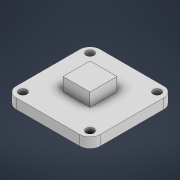
# Autodesk Inventor part: camera
Saved by Autodesk Inventor 2021 (Build 250183000, 183)
## iProperties
Created: 2020-12-29
Part Number: camera
Material: Generic
Document SubType Name: Modeling
Designer: Tomasz
Density: 1 g/cm^3
Appearance: Default
Author: Tomasz
Autodesk Inventor part; units mm, degrees
ref_plane "YZ Plane" through (0, 0, 0) normal (1, 0, 0) x (0, 1, 0)
ref_plane "XZ Plane" through (0, 0, 0) normal (0, 1, 0) x (-1, 0, 0)
ref_plane "XY Plane" through (0, 0, 0) normal (0, 0, 1) x (1, 0, 0)
sketch "Sketch1" plane through (0, 0, 0) normal (0, 1, 0) x (-1, 0, 0)
  line L0 (-9.5, 12.5) -> (9.5, 12.5)
  line L1 (12.5, 9.5) -> (12.5, -9.5)
  line L2 (9.5, -12.5) -> (-9.5, -12.5)
  line L3 (-12.5, -9.5) -> (-12.5, 9.5)
  line L4 (-12.5, 12.5) -> (12.5, -12.5) construction
  line L5 (12.5, 12.5) -> (-12.5, -12.5) construction
  line L6 (-10, -10) -> (10, -10) construction
  line L7 (10, -10) -> (10, 10) construction
  line L8 (10, 10) -> (-10, 10) construction
  line L9 (-10, 10) -> (-10, -10) construction
  line L10 (-10, -10) -> (10, 10) construction
  line L11 (10, -10) -> (-10, 10) construction
  circle A0 centre (10, 10) radius 1.2
  circle A1 centre (10, -10) radius 1.2
  circle A2 centre (-10, 10) radius 1.2
  circle A3 centre (-10, -10) radius 1.2
  arc A4 (12.5, 9.5) -> (9.5, 12.5) centre (9.5, 9.5) ccw
  arc A5 (9.5, -12.5) -> (12.5, -9.5) centre (9.5, -9.5) ccw
  arc A6 (-9.5, 12.5) -> (-12.5, 9.5) centre (-9.5, 9.5) ccw
  arc A7 (-12.5, -9.5) -> (-9.5, -12.5) centre (-9.5, -9.5) ccw
  point P0 (0, 0)
  dimension "d0" = 25
  dimension "d1" = 25
  dimension "d2" = 20
  dimension "d3" = 20
  dimension "d4" = 2.4
  dimension "d7" = 20
  dimension "d10" = 20
  dimension "d13" = 3
  constraints: 24 end point, 8 centre point, 8 point on circle, 8 point on line, 8 tangent, 4 midpoint, 4 parallel, 3 equal radius, 3 horizontal, 2 perpendicular, 1 coincident, 1 vertical, 6 other
  measures "d0" distance of L4.end L5.end
  measures "d1" distance of L5.start L4.end
  measures "d2" distance of L8.end L7.end
  measures "d3" distance of L7.end L6.end
  measures "d4" diameter of A0
  measures "d7" distance of A0.centre A1.centre
  measures "d10" distance of A0.centre A2.centre
  measures "d13" radius of A4
extrude "Extrusion1" add sketch "Sketch1" along normal blind 3
sketch "Sketch2" plane through (0, 3, 0) normal (0, 1, 0) x (1, 0, 0)
  line L0 (4, -4) -> (-4, -4)
  line L1 (-4, -4) -> (-4, 4)
  line L2 (-4, 4) -> (4, 4)
  line L3 (4, 4) -> (4, -4)
  line L4 (4, -4) -> (-4, 4) construction
  line L5 (-4, -4) -> (4, 4) construction
  point P0 (0, 0)
  dimension "d16" = 8
  dimension "d17" = 8
  constraints: 12 end point, 2 midpoint, 2 parallel, 1 horizontal, 1 perpendicular
  measures "d16" distance of L1.end L2.end
  measures "d17" distance of L0.end L1.end
extrude "Extrusion2" add sketch "Sketch2" along normal blind 3.98
equation "\"d4\" = hole"
equation "\"hole\" = 2.4"
body "Solid1"
